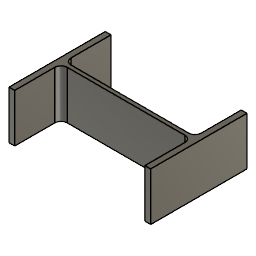
H-294×200×8×12 (Autodesk Fusion 360 design; units mm, degrees)
Autodesk Fusion 360 part; units mm, degrees
sketch "スケッチ1" plane through (0, 0, 0) normal (0, 0, 1) x (1, 0, 0)
  line L0 (0, 100) -> (0, -100)
  line L1 (12, 17) -> (12, 100)
  line L2 (282, 100) -> (282, 17)
  line L3 (294, -100) -> (294, 100)
  line L4 (282, -17) -> (282, -100)
  line L5 (12, -100) -> (12, -17)
  line L6 (0, -100) -> (12, -100)
  line L7 (282, -100) -> (294, -100)
  line L8 (269, 4) -> (25, 4)
  line L9 (25, -4) -> (269, -4)
  line L10 (12, 100) -> (0, 100)
  line L11 (294, 100) -> (282, 100)
  arc A0 (25, -4) -> (12, -17) centre (25, -17) ccw
  arc A1 (12, 17) -> (25, 4) centre (25, 17) ccw
  arc A2 (269, 4) -> (282, 17) centre (269, 17) ccw
  arc A3 (282, -17) -> (269, -4) centre (269, -17) ccw
extrude "押し出し1" add sketch "スケッチ1" along normal blind 100
